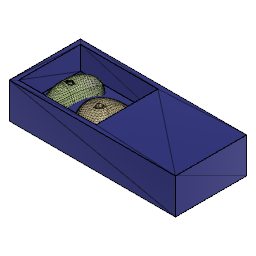
Assignment6_final (Autodesk Fusion 360 design; units mm, degrees)
Autodesk Fusion 360 part; units mm, degrees
note: some values were not read from the file. Chosen so that the rebuilt part matches the saved one: that a step has no effect.
sketch "Sketch1" plane through (0, 0, 0) normal (0, 0, 1) x (1, 0, 0)
  line L0 (0, 0) -> (177.8, 0)
  line L1 (177.8, 0) -> (177.8, 76.2)
  line L2 (177.8, 76.2) -> (0, 76.2)
  line L3 (0, 76.2) -> (0, 0)
  dimension "d1" = 177.8
  dimension "d2" = 76.2
  constraint horizontal L0
  constraint vertical L1
  constraint horizontal L2
  constraint vertical L3
  constraint coincident L0.start L3.end
  measures "d1" distance of L0.start L0.end
  measures "d2" distance of L0.start L2.end
extrude "Extrude1" add sketch "Sketch1" along normal blind 38.1
sketch "Sketch2" plane through (0, 0, 38.1) normal (0, 0, 1) x (-1, 0, 0)
  line L0 (0, -76.2) -> (0, 0)
  line L1 (0, 0) -> (-177.8, 0)
  line L2 (-177.8, 0) -> (-177.8, -76.2)
  line L3 (-177.8, -76.2) -> (0, -76.2)
  line L4 (-5, -5) -> (-87.8, -5)
  line L5 (-87.8, -5) -> (-87.8, -71.2)
  line L6 (-87.8, -71.2) -> (-5, -71.2)
  line L7 (-5, -71.2) -> (-5, -5)
  dimension "d5" = 5
  dimension "d6" = 5
  dimension "d7" = 5
  dimension "d8" = 90
  constraint horizontal L4
  constraint vertical L5
  constraint horizontal L6
  constraint vertical L7
  measures "d5" distance of L3 L6
  measures "d6" distance of L0 L7
  measures "d7" distance of L1 L4
  measures "d8" distance of L2 L5
extrude "Extrude2" cut sketch "Sketch2" against normal blind 25 contours L4 L5 L6 L7
mesh "Mesh6" [no effect]
mesh "Mesh7" [no effect]
mesh "Mesh8" [no effect]
mesh "Mesh9" [no effect]
form "Form1" [no effect]
mesh "Mesh10" [no effect]
mesh "Mesh11" [no effect]
